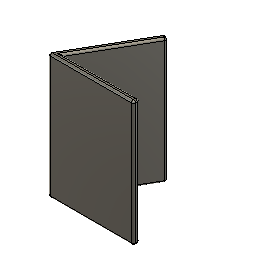
SeMaSHolder (Autodesk Fusion 360 design; units mm, degrees)
Autodesk Fusion 360 part; units mm, degrees
sketch "Sketch1" plane through (0, 0, 0) normal (0, 1, 0) x (1, 0, 0)
  line L0 (0, 0) -> (22.5, 38.9711)
  line L1 (0, 0) -> (45, 0) construction
  line L2 (22.5, 38.9711) -> (25.0981, 37.4711)
  line L3 (22.5, 38.9711) -> (25.5, 38.9711) construction
  line L4 (25.0981, 37.4711) -> (3.4641, 0)
  line L5 (25.0981, 37.4711) -> (68.366, 37.4711) construction
  line L6 (0, 0) -> (45, 0)
  line L7 (45, 0) -> (45, 3)
  line L8 (45, 3) -> (1.7321, 3)
  dimension "d1" = 45
  dimension "d2" = 60
  dimension "d3" = 30
  dimension "d4" = 3
  dimension "d5" = 120
  dimension "d6" = 45
  dimension "d7" = 3
  constraint horizontal L1
  constraint coincident L0.start L1.start
  constraint horizontal L3
  constraint horizontal L5
  constraint coincident L1 L4.end
  constraint perpendicular L6 L7
  constraint coincident L0 L8.end
  constraint perpendicular L7 L8
  measures "d1" distance of L0.start L0.end
  measures "d2" angle of L0 L1
  measures "d3" angle of L2 L3
  measures "d4" distance of L0.end L2.end
  measures "d5" angle of L4 L5
  measures "d6" distance of L1.end L0.start
  measures "d7" distance of L1.end L7.end
extrude "Extrude1" add sketch "Sketch1" along normal blind 45
extrude "Extrude2" add 1 faces at (9.8094, 45, -14.9904) along direction (0, 1, 0) blind 20
fillet "Fillet1" radius 1 17 edges at (0, 32.5, 0) (22.5, 32.5, -38.9711) (11.25, 65, -19.4856) (11.25, 0, -19.4856) (22.5, 0, 0) (45, 32.5, 0) (22.5, 65, 0) (15.1471, 65, -20.2356) (25.0981, 65, -3) (15.1471, 0, -20.2356) (25.0981, 0, -3) (25.0981, 32.5, -37.4711) (23.799, 65, -38.2211) (23.799, 0, -38.2211) (45, 65, -1.5) (45, 32.5, -3) (45, 0, -1.5)
